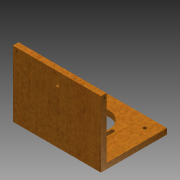
# Autodesk Inventor part: frame_fixed
Saved by Autodesk Inventor 2014 (Build 180170000, 170)
## iProperties
Created: 2015-01-04
Part Number: frame_fixed
Material: Generic
Document SubType Name: Modeling
Designer: cruiser
Density: 1 g/cm^3
Appearance: Yellow Pine - Solid Stained Light Low Gloss
Author: cruiser
Autodesk Inventor part; units mm, degrees
ref_plane "YZ Plane" through (0, 0, 0) normal (1, 0, 0) x (0, 1, 0)
ref_plane "XZ Plane" through (0, 0, 0) normal (0, 1, 0) x (-1, 0, 0)
ref_plane "XY Plane" through (0, 0, 0) normal (0, 0, 1) x (1, 0, 0)
sketch "Sketch1" plane through (0, 0, 0) normal (0, 0, 1) x (1, 0, 0)
  line L0 (40, -30) -> (-40, -30)
  line L1 (-40, -30) -> (-40, 30)
  line L2 (-40, 30) -> (40, 30)
  line L3 (40, 30) -> (40, -30)
  line L4 (40, -30) -> (-40, 30) construction
  line L5 (-40, -30) -> (40, 30) construction
  circle A0 centre (0, 0) radius 14.5
  circle A1 centre (-17.5, 0) radius 1.575
  line L6 (0, 0) -> (-17.5, 0)
  circle A2 centre (17.5, 0) radius 1.575
  line L7 (0, 0) -> (0, -14.5)
  line L8 (-10, -20) -> (-10, 0)
  line L9 (-10, 0) -> (10, 0)
  line L10 (10, 0) -> (10, -20)
  line L11 (10, -20) -> (-10, -20)
  line L12 (-10, -20) -> (10, 0) construction
  line L13 (-10, 0) -> (10, -20) construction
  circle A3 centre (-30, 20) radius 1.575
  circle A4 centre (30, 20) radius 1.575
  circle A5 centre (-30, -20) radius 1.575
  circle A6 centre (30, -20) radius 1.575
  point P0 (0, -10)
  dimension "d6" = 29
  dimension "d0" = 3.15
  dimension "d1" = 17.5
  dimension "d4" = 360
  dimension "d7" = 20
  dimension "d8" = 20
  dimension "d9" = 60
  dimension "d10" = 80
  dimension "d13" = 3.15
  dimension "d14" = 10
  dimension "d15" = 10
  constraints: 28 end point, 6 centre point, 5 parallel, 4 midpoint, 4 perpendicular, 3 symmetric about line, 1 coincident, 1 collinear, 1 horizontal, 1 point on line, 1 vertical alignment, 10 other
  measures "d0" diameter of A1
  measures "d1" distance of L6.start L6.end
  measures "d7" distance of L10.end L8.start
  measures "d8" distance of L9.end L10.end
  measures "d9" distance of L2.end L0.start
  measures "d10" distance of L1.end L2.end
  measures "d13" diameter of A3
  measures "d14" distance from line of L2 A3.centre
  measures "d15" distance from line of L1 A3.centre
extrude "Extrusion1" add sketch "Sketch1" along normal blind 5.08
sketch "Sketch3" plane through (0, 0, 5.08) normal (0, 0, 1) x (1, 0, 0)
  arc A0 (10, -10.5) -> (-10, -10.5) centre (0, 0) ccw projected
  line L0 (10, -10.5) -> (10, -20) projected
  circle A1 centre (17.5, 0) radius 1.575 projected
  circle A2 centre (-17.5, 0) radius 1.575 projected
  line L1 (40, 30) -> (-40, 30) projected
  line L2 (-17.5, -3) -> (-17.5, 3) construction
  line L3 (-15.925, -3) -> (-15.925, 3)
  line L4 (-19.075, 3) -> (-19.075, -3)
  arc A3 (-19.075, -3) -> (-15.925, -3) centre (-17.5, -3) ccw
  arc A4 (-15.925, 3) -> (-19.075, 3) centre (-17.5, 3) ccw
  line L5 (0, 0) -> (0, 30)
  line L6 (15.925, -3) -> (15.925, 3)
  line L7 (19.075, 3) -> (19.075, -3)
  arc A5 (15.925, -3) -> (19.075, -3) centre (17.5, -3) ccw
  arc A6 (19.075, 3) -> (15.925, 3) centre (17.5, 3) ccw
  line L8 (0, -3) -> (0, 3) construction
  line L9 (14.5, -3) -> (14.5, 3)
  line L10 (-14.5, 3) -> (-14.5, -3)
  arc A7 (-14.5, -3) -> (14.5, -3) centre (0, -3) ccw
  arc A8 (14.5, 3) -> (-14.5, 3) centre (0, 3) ccw
  line L11 (-10, -20) -> (10, -20)
  line L12 (10, -20) -> (10, -23)
  line L13 (10, -23) -> (-10, -23)
  line L14 (-10, -23) -> (-10, -20)
  dimension "d20" = 3
  dimension "d21" = 1.575
  dimension "d22" = 3
  dimension "d23" = 0
  dimension "d24" = 3
  constraints: 30 end point, 12 point on circle, 8 tangent, 6 centre point, 6 symmetric about line, 5 parallel, 3 midpoint, 1 collinear, 1 horizontal, 1 perpendicular, 1 point on line, 2 other
  measures "d20" distance of A2.centre L2.end
  measures "d21" radius of A4
  measures "d22" distance of L5.start L8.end
  measures "d23" distance edge to line of A0 L9
  measures "d24" distance of L11.end L12.end
extrude "Extrusion3" cut sketch "Sketch3" against normal blind 10 contours L0 A7 L10 A0 | A0 L9 A7 L0 | A0 L5 A8 L9 | A0 L10 A8 L5 | L7 A5 L6 A1 | A1 L6 A6 L7 | L3 A3 L4 A2 | A2 L4 A4 L3 | L11 L12 L13 L14
sketch "Sketch5" plane through (0, 0, 5.08) normal (0, 0, 1) x (1, 0, 0)
  line L0 (-40, -30) -> (40, -30) projected
  line L1 (40, -30) -> (40, 30) projected
  line L2 (-40, -30) -> (40, -30)
  line L3 (40, -30) -> (40, -24.92)
  line L4 (40, -24.92) -> (-40, -24.92)
  line L5 (-40, -24.92) -> (-40, -30)
  point P0 (0, 0)
  dimension "d30" = 5.08
  constraints: 8 end point, 2 parallel, 1 horizontal, 1 perpendicular, 1 point on line
  measures "d30" distance between parallel lines of L2 L4
extrude "Extrusion5" add sketch "Sketch5" along normal blind 55
sketch "Sketch6" plane through (-40, -24.92, 5.08) normal (0, 1, 0) x (1, 0, 0)
  line L0 (0, 0) -> (80, 0) projected
  line L1 (80, -55) -> (0, -55) projected
  line L2 (40, 0) -> (40, -55)
  circle A0 centre (40, -43.8) radius 1.575
  point P0 (40, 5.08)
  dimension "d33" = 3.15
  dimension "d34" = 43.8
  constraints: 2 end point, 2 midpoint, 1 centre point, 1 point on line
  measures "d33" diameter of A0
  measures "d34" distance from line of L0 A0.centre
extrude "Extrusion6" cut sketch "Sketch6" against normal blind 50
sketch "Sketch4" plane through (0, 0, 5.08) normal (0, 0, 1) x (1, 0, 0)
  line L0 (-40, -30) -> (40, -30) projected
  line L1 (40, 30) -> (34.92, 30)
  line L2 (34.92, 30) -> (34.92, -30)
  line L3 (34.92, -30) -> (40, -30)
  line L4 (40, -30) -> (40, 30)
  point P0 (0, 0)
  dimension "d27" = 5.08
  constraints: 8 end point, 2 parallel, 1 horizontal, 1 perpendicular, 1 point on line
  measures "d27" distance between parallel lines of L4 L2
equation "\"d0\" = m3_diameter"
equation "\"d1\" = 0.5 * stepper_screw_space"
equation "\"d13\" = m3_diameter"
equation "\"d11\" = wood_thickness"
equation "\"d21\" = 0.5 * m3_diameter"
equation "\"d30\" = wood_thickness"
equation "\"d33\" = m3_diameter"
equation "\"d27\" = wood_thickness"
equation "\"wood_thickness\" = 5.08"
equation "\"m5_diameter\" = 5.25"
equation "\"m3_diameter\" = 3.15"
equation "\"stepper_screw_space\" = 35"
equation "\"stepper_body_diameter\" = 28"
equation "\"stepper_shaft_diameter\" = 5"
equation "\"laser_body_diameter\" = 12"
body "Solid1"
body "Solid2"
